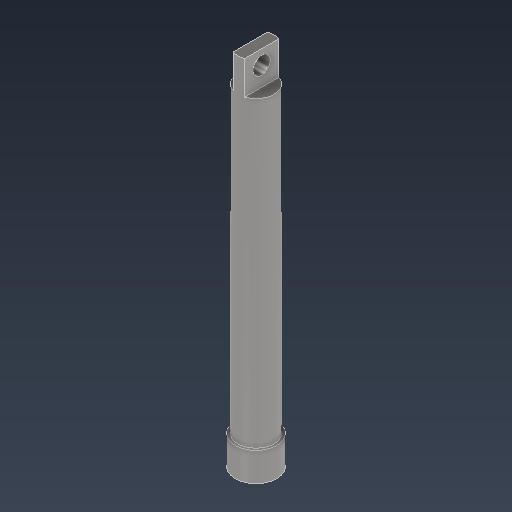
# Autodesk Inventor part: SP6V1 Vastago Freno
Saved by Autodesk Inventor 2021.2 (Build 252289000, 289)
## iProperties
Created: 2026-06-23
Part Number: SP6V1 Vastago Freno
Material: Stainless Steel
Document SubType Name: Modeling
Designer: nelso
Density: 8.08 g/cm^3
Appearance: Semi-Polished
Mass: 123.244 g
Surface Area: 53.4821 cm^2
Volume: 15.2529 cm^3
Author: nelso
Autodesk Inventor part; units mm, degrees
ref_plane "YZ Plane" through (0, 0, 0) normal (1, 0, 0) x (0, 1, 0)
ref_plane "XZ Plane" through (0, 0, 0) normal (0, 1, 0) x (-1, 0, 0)
ref_plane "XY Plane" through (0, 0, 0) normal (0, 0, 1) x (1, 0, 0)
sketch "Sketch1" plane through (0, 0, 0) normal (0, 1, 0) x (-1, 0, 0)
  circle A0 centre (0, 0) radius 6.3
  dimension "d0" = 12.6
  constraints: 1 centre point, 1 coincident
  measures "d0" diameter of A0
extrude "Extrusion1" add sketch "Sketch1" along normal mid plane 127
sketch "Sketch2" plane through (0, 0, 0) normal (1, 0, 0) x (0, 1, 0)
  line L0 (63.5, -6.3) -> (63.5, 6.3) projected
  line L1 (-63.5, -6.3) -> (63.5, -6.3) projected
  line L2 (63.5, 6.3) -> (51.87, 6.3)
  line L3 (51.87, 6.3) -> (51.87, -6.3)
  line L4 (51.87, -6.3) -> (63.5, -6.3)
  line L5 (63.5, -6.3) -> (63.5, 6.3)
  line L6 (63.5, 0) -> (58.5, 0)
  circle A0 centre (58.5, 0) radius 3
  point P0 (0, 0)
  dimension "d3" = 11.63
  dimension "d7" = 5
  dimension "d8" = 6
  constraints: 10 end point, 2 horizontal, 2 parallel, 1 centre point, 1 coincident, 1 midpoint, 1 perpendicular, 1 point on line
  measures "d3" distance of L4.end L3.end
  measures "d7" distance of L6.start L6.end
  measures "d8" diameter of A0
sketch "Sketch3" plane through (0, 63.5, 0) normal (0, 1, 0) x (1, 0, 0)
  circle A0 centre (0, 0) radius 6.3 projected
  line L0 (2, -5.9741) -> (-2, -5.9741)
  line L1 (-2, -5.9741) -> (-2, 5.9741)
  line L2 (-2, 5.9741) -> (2, 5.9741)
  line L3 (2, 5.9741) -> (2, -5.9741)
  line L4 (2, -5.9741) -> (-2, 5.9741) construction
  line L5 (-2, -5.9741) -> (2, 5.9741) construction
  dimension "d4" = 4
  constraints: 12 end point, 2 midpoint, 2 parallel, 1 horizontal, 1 perpendicular, 1 point on circle
  measures "d4" distance of L1.end L2.end
extrude "Extrusion2" cut sketch "Sketch3" against normal blind 11.63 contours A0 L3 | L1 A0
extrude "Extrusion3" cut sketch "Sketch2" against normal mid plane 11.63 contours A0
sketch "Sketch4" plane through (0, -63.5, 0) normal (0, -1, 0) x (1, 0, 0)
  circle A0 centre (0, 0) radius 7.25
  dimension "d11" = 14.5
  constraints: 1 centre point, 1 coincident
  measures "d11" diameter of A0
extrude "Extrusion4" add sketch "Sketch4" against normal blind 10
body "Solid1"
